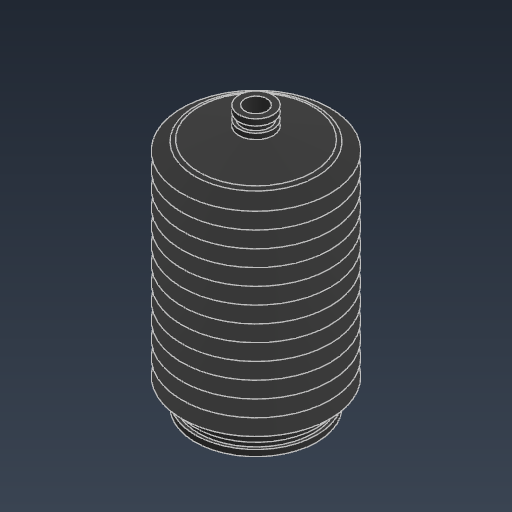
# Autodesk Inventor part: MCEN4000:T7
Saved by Autodesk Inventor 2021 (Build 250183000, 183)
## iProperties
Created: 2020-10-22
Part Number: MCEN4000:T7
Material: RUBBER, SILICONE
Document SubType Name: Modeling
Designer: Tang Kang Ning
Mass: 98.3912 g
Surface Area: 1566.54 cm^2
Volume: 87.8492 cm^3
Density: 1.12 g/cm^3
Appearance: Rubber - Black
Description: BALL JOINT BELLOW
Author: Tang Kang Ning
Autodesk Inventor part; units mm, degrees
ref_plane "YZ Plane" through (0, 0, 0) normal (1, 0, 0) x (0, 1, 0)
ref_plane "XZ Plane" through (0, 0, 0) normal (0, 1, 0) x (-1, 0, 0)
ref_plane "XY Plane" through (0, 0, 0) normal (0, 0, 1) x (1, 0, 0)
sketch "Sketch2" plane through (0, 0, 0) normal (0, 0, 1) x (1, 0, 0)
  line L0 (-9, 221.1144) -> (9, 221.1144) projected
  line L1 (37, 65.25) -> (-37, 65.25) projected
  point P0 (0, 0)
  dimension "d38" = 155.8644
  measures "d38" distance between parallel lines of L0 L1
sketch "Sketch1" plane through (0, 0, 0) normal (0, 0, 1) x (1, 0, 0)
  line L0 (-36.7449, 53.25) -> (37.2551, 53.25)
  line L1 (35, 65.25) -> (35, 53.25)
  line L2 (7, 221.1144) -> (7, 209.1144)
  line L3 (7, 221.1144) -> (7, 209.1144)
  line L4 (7, 221.1144) -> (11, 221.1144)
  line L5 (35, 53.25) -> (39, 53.25)
  line L6 (39, 53.25) -> (39, 57.25)
  line L7 (39, 57.25) -> (37, 57.25)
  line L8 (37, 57.25) -> (37, 61.25)
  line L9 (37, 61.25) -> (39, 61.25)
  line L10 (39, 61.25) -> (39, 65.25)
  line L11 (39, 65.25) -> (37, 65.25) construction
  line L12 (11, 221.1144) -> (11, 217.1144)
  line L13 (11, 217.1144) -> (9, 217.1144)
  line L14 (9, 217.1144) -> (9, 213.1144)
  line L15 (9, 213.1144) -> (11, 213.1144)
  line L16 (11, 213.1144) -> (11, 209.5606)
  line L17 (39, 65.25) -> (47.5328, 70.4646)
  line L18 (37, 65.25) -> (45.5328, 70.4646)
  line L19 (37, 65.25) -> (37, 83.6946) construction
  line L20 (45.5328, 70.4646) -> (37, 70.4646) construction
  line L21 (45.5328, 70.4646) -> (37, 75.6791)
  line L22 (47.5328, 70.4646) -> (39, 75.6791)
  line L23 (37, 75.6791) -> (46.5513, 75.6791) construction
  line L24 (45.5328, 80.8937) -> (37, 86.1083)
  line L25 (47.5328, 80.8937) -> (39, 86.1083)
  line L26 (39, 75.6791) -> (47.5328, 80.8937)
  line L27 (37, 75.6791) -> (45.5328, 80.8937)
  line L28 (45.5328, 91.3228) -> (37, 96.5374)
  line L29 (47.5328, 91.3228) -> (39, 96.5374)
  line L30 (39, 86.1083) -> (47.5328, 91.3228)
  line L31 (37, 86.1083) -> (45.5328, 91.3228)
  line L32 (45.5328, 101.752) -> (37, 106.9665)
  line L33 (47.5328, 101.752) -> (39, 106.9665)
  line L34 (39, 96.5374) -> (47.5328, 101.752)
  line L35 (37, 96.5374) -> (45.5328, 101.752)
  line L36 (45.5328, 112.1811) -> (37, 117.3956)
  line L37 (47.5328, 112.1811) -> (39, 117.3956)
  line L38 (39, 106.9665) -> (47.5328, 112.1811)
  line L39 (37, 106.9665) -> (45.5328, 112.1811)
  line L40 (45.5328, 122.6102) -> (37, 127.8248)
  line L41 (47.5328, 122.6102) -> (39, 127.8248)
  line L42 (39, 117.3956) -> (47.5328, 122.6102)
  line L43 (37, 117.3956) -> (45.5328, 122.6102)
  line L44 (45.5328, 133.0393) -> (37, 138.2539)
  line L45 (47.5328, 133.0393) -> (39, 138.2539)
  line L46 (39, 127.8248) -> (47.5328, 133.0393)
  line L47 (37, 127.8248) -> (45.5328, 133.0393)
  line L48 (45.5328, 143.4685) -> (37, 148.683)
  line L49 (47.5328, 143.4685) -> (39, 148.683)
  line L50 (39, 138.2539) -> (47.5328, 143.4685)
  line L51 (37, 138.2539) -> (45.5328, 143.4685)
  line L52 (45.5328, 153.8976) -> (37, 159.1122)
  line L53 (47.5328, 153.8976) -> (39, 159.1122)
  line L54 (39, 148.683) -> (47.5328, 153.8976)
  line L55 (37, 148.683) -> (45.5328, 153.8976)
  line L56 (45.5328, 164.3267) -> (37, 169.5413)
  line L57 (47.5328, 164.3267) -> (39, 169.5413)
  line L58 (39, 159.1122) -> (47.5328, 164.3267)
  line L59 (37, 159.1122) -> (45.5328, 164.3267)
  line L60 (45.5328, 174.7559) -> (37, 179.9704)
  line L61 (47.5328, 174.7559) -> (39, 179.9704)
  line L62 (39, 169.5413) -> (47.5328, 174.7559)
  line L63 (37, 169.5413) -> (45.5328, 174.7559)
  line L64 (45.5328, 185.185) -> (37, 190.3996)
  line L65 (47.5328, 185.185) -> (39, 190.3996)
  line L66 (39, 179.9704) -> (47.5328, 185.185)
  line L67 (37, 179.9704) -> (45.5328, 185.185)
  line L68 (0, -37.6229) -> (0, 264.2373)
  line L69 (9, 209.1144) -> (7, 209.1144)
  line L70 (37, 65.25) -> (35, 65.25)
  line L71 (0, 208431.7305) -> (0, -209414.2305)
  line L72 (37, 65.25) -> (-37, 65.25) projected
  line L73 (37, 65.25) -> (-37, 65.25) construction
  line L74 (-9, 209.1144) -> (9, 209.1144) projected
  line L75 (37, 65.25) -> (35, 65.25)
  line L76 (7, 209.1144) -> (9, 209.1144)
  line L77 (9, 209.1144) -> (37.2519, 200.6748)
  line L78 (11, 209.5606) -> (36.5024, 201.9423)
  arc A0 (39, 200.8287) -> (36.5024, 201.9423) centre (33.4633, 191.7688) ccw
  line L79 (-9, 209.1144) -> (9, 209.1144) projected
  line L80 (45.5328, 195.6141) -> (37, 200.8287)
  line L81 (47.5328, 195.6141) -> (39, 200.8287)
  line L82 (39, 190.3996) -> (47.5328, 195.6141)
  line L83 (37, 190.3996) -> (45.5328, 195.6141)
  point P0 (0, 0)
  point P1 (11, 206.3274)
  point P2 (39, 75.6791)
  point P3 (7, 203.6144)
  point P4 (39, 200.8287)
  dimension "d0" = 4
  dimension "d1" = 12
  dimension "d2" = 4
  dimension "d3" = 2
  dimension "d4" = 2
  dimension "d5" = 4
  dimension "d7" = 2
  dimension "d8" = 2
  dimension "d12" = 121.43
  dimension "d13" = 1.0429
  dimension "d17" = 10
  dimension "d18" = 10.4291
  dimension "d28" = 10.4291
  dimension "d34" = 12
  dimension "d37" = 7
  dimension "d39" = 155.8644
  dimension "d42" = 4
  dimension "d44" = 106.632
  dimension "d45" = 1
  dimension "d46" = 2
  constraints: 160 end point, 13 perpendicular, 9 point on line, 5 vertical, 3 horizontal, 3 parallel, 2 coincident, 2 collinear, 2 point on circle, 2 tangent, 1 centre point, 1 equal length, 124 other
  measures "d0" distance between parallel lines of L11 L9
  measures "d1" distance of L1.start L1.end
  measures "d2" distance between parallel lines of L5 L7
  measures "d3" distance between parallel lines of L8 L10
  measures "d4" distance between parallel lines of L1 L8
  measures "d5" distance of L4.end L12.end
  measures "d7" distance between parallel lines of L2 L14
  measures "d8" distance between parallel lines of L14 L16
  measures "d12" angle of L10 L17
  measures "d13" distance between parallel lines of L17 L18
  measures "d17" distance of L10.end L17.end
  measures "d18" distance of L11.end L21.end
  measures "d28" distance of L18.end L24.start
  measures "d34" distance of L2.end L2.start
  measures "d37" distance between parallel lines of L2 L68
  measures "d39" distance between parallel lines of L69 L0
  measures "d42" distance between parallel lines of L15 L74
  measures "d44" angle of L16 L77
  measures "d45" distance between parallel lines of L78 L77
  measures "d46" distance of L2.end L69.start
revolve "Revolution1" add sketch "Sketch1" angle 360 about axis through (0, -37.6229, 0) along (0, 1, 0) contours L1 L70 L18 L21 L27 L24 L31 L28 L35 L32 L39 L36 L43 L40 L47 L44 L51 L48 L55 L52 L59 L56 L63 L60 L67 L64 L83 L80 L77 L69 L2 L4 L12 L13 L14 L15 L16 L78 A0 L81 L82 L65 L66 L61 L62 L57 L58 L53 L54 L49 L50 L45 L46 L41 L42 L37 L38 L33 L34 L29 L30 L25 L26 L22 L17 L10 L9 L8 L7 L6 L5 L0
equation "\"d0\" = 0.333333 * d1"
equation "\"d2\" = d0"
equation "\"d5\" = d0"
equation "\"d28\" = d18"
equation "\"d37\" = RevolveDIA"
equation "\"d39\" = d38"
equation "\"d42\" = d5"
equation "\"d44\" = d38_1"
equation "\"d10\" = d9"
equation "\"RevolveDIA\" = 7"
equation "\"d38_1\" = 106.632348deg"
equation "\"d9\" = 171.191599"
body "Solid1"
